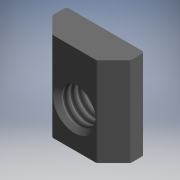
# Autodesk Inventor part: 25-1964
Saved by Autodesk Inventor 2017.3 (Build 213256000, 256)
## iProperties
Part Number: 25-1964
Material: Generic
Catalog Web Link: www.cadenas.de
Description: 25-1954, 25-1964, 25-3204, 25-8901, 40-1964, 40-1984, 40-3202, 40-3203, 40-8900-Slide-In T-Nuts
Vendor: 8020
Document SubType Name: Modeling
Designer: partserver
Manufacturer: 8020
Mass: 0.432501 g
Surface Area: 4.44508 cm^2
Volume: 0.432501 cm^3
Density: 1 g/cm^3
Appearance: PSOLRGB-127-127-127
Category: PARTsolutions
Company: 8020
Title: 25-1964
Author: Cadenas PARTsolutions
Comments: Slide-In T-Nuts
PSOL_IDENT_0: {$CADENAS_DATA\23d-libs\8020\metric\fastening_options\25_1954.prj},227 {VTYP=3D},{NB=25-1964},{LINA=
PSOL_IDENT_1: 25-1964},{NN=25-1954, 25-1964, 25-3204, 25-8901, 40-1964, 40-1984, 40-3202, 40-3203, 40-8900},{DATE=
PSOL_IDENT_2: 31.07.2020 09:21:26},{GEOMDATE=15.05.2012 11:39:00},{VERSION=},{LINEID=30},{WBVAR=},{WBNUMERIC=}  {N
PSOL_IDENT_3: B=25-1964},{LINA=25-1964},{KT=DUMMY},{PN=25-1964},{MAT=1215 Carbon Steel},{FIN=Bright Zinc},{A=4.34}
PSOL_IDENT_4: ,{A1=4.34340},{B=5.08},{B1=5.08000},{C=12.45},{C1=12.44600},{D=10.95},{D1=10.94740},{E=M6 x 1.0},{E1=
PSOL_IDENT_5: 6.00000},{TT=M},{W=.0045},{COL=0.50,0.50,0.50,0.00},{NO=2}
NB: 25-1964
NN: 25-1954, 25-1964, 25-3204, 25-8901, 40-1964, 40-1984, 40-3202, 40-3203, 40-8900
NT: Slide-In T-Nuts
NBSYN: $PN.
LINA: 25-1964
CATALOG: 80/20
PN: 25-1964
MAT: 1215 Carbon Steel
FIN: Bright Zinc
A: 4.34
B: 5.08
C: 12.45
D: 10.95
E: M6 x 1.0
W: .0045
SUPPLIER: 8020
ARTICLENO: 25-1964
BOMINFO: 25-1964
CREATOR: CADENAS GmbH
Autodesk Inventor part; units mm, degrees
sketch "Sketch_1" plane through (0, 0, -7.366) normal (0, 0, 1) x (1, 0, 0)
  line L0 (-5.4737, 3.9624) -> (-5.4737, 2.5467)
  arc A0 (-5.4737, 2.5467) -> (-5.3621, 2.2773) centre (-5.0927, 2.5467) ccw
  line L1 (-5.3621, 2.2773) -> (-3.1964, 0.1116)
  arc A1 (-3.1964, 0.1116) -> (-2.927, 0) centre (-2.927, 0.381) ccw
  line L2 (-2.927, 0) -> (2.927, 0)
  arc A2 (2.927, 0) -> (3.1964, 0.1116) centre (2.927, 0.381) ccw
  line L3 (3.1964, 0.1116) -> (5.3621, 2.2773)
  arc A3 (5.3621, 2.2773) -> (5.4737, 2.5467) centre (5.0927, 2.5467) ccw
  line L4 (5.4737, 2.5467) -> (5.4737, 3.9624)
  arc A4 (5.4737, 3.9624) -> (5.0927, 4.3434) centre (5.0927, 3.9624) ccw
  line L5 (5.0927, 4.3434) -> (-5.0927, 4.3434)
  arc A5 (-5.0927, 4.3434) -> (-5.4737, 3.9624) centre (-5.0927, 3.9624) ccw
  constraints: 12 end point, 12 point on circle, 6 centre point
extrude "Extrusion1" add sketch "Sketch_1" along normal blind 12.446
sketch "Sketch_4" plane through (0, 0, 0) normal (0, 0, 1) x (1, 0, 0)
  line L0 (0, 0) -> (0, 4.3434)
  line L1 (0, 4.3434) -> (3, 4.3434)
  line L2 (3, 4.3434) -> (2.4585, 3.8019)
  line L3 (2.4585, 3.8019) -> (2.4585, 0.5415)
  line L4 (2.4585, 0.5415) -> (3, 0)
  line L5 (3, 0) -> (0, 0)
  line L6 (0, 0) -> (0, 4.3434)
  constraints: 14 end point
revolve "Revolution1" cut sketch "Sketch_4" angle 360 about axis through (0, 0, 0) along (0, -1, 0)
thread "Thread1" size "M6x1" class "6H" standard "ISO Metric profile" full length
ref_plane "tnut_XY" through (0, 4.3434, 0) normal (0, 1, 0) x (1, 0, 0)
ref_plane "tnut_YZ" through (0, 4.3434, 0) normal (1, 0, 0) x (0, 0, -1)
ref_plane "tnut_ZX" through (0, 4.3434, 0) normal (0, 0, -1) x (0, 1, 0)
body "Solid1"
